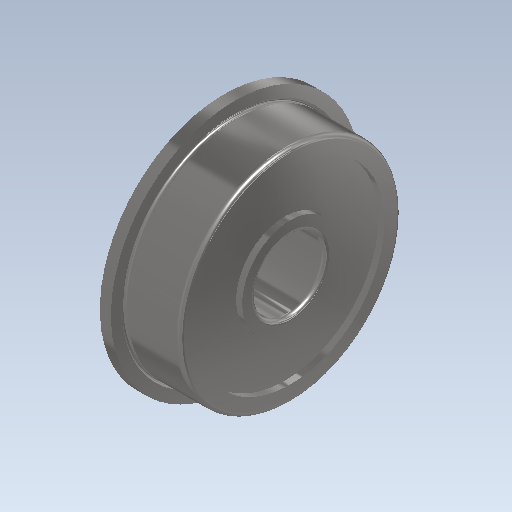
# Autodesk Inventor part: flange-bearing
Saved by Autodesk Inventor 2020 (Build 240168000, 168)
## iProperties
Part Number: flange-bearing
Material: Stainless Steel, 440C
Catalog Web Link: www.cadenas.de
Description: SFLC6 _ _ ZZ-Low Dust Raise Greased Ball Bearings - Double Shielded with Flange
Vendor: MISUMI
Document SubType Name: Modeling
Designer: partserver
Manufacturer: MISUMI
Mass: 12.691 g
Surface Area: 13.427 cm^2
Volume: 1.63755 cm^3
Density: 7.75 g/cm^3
Appearance: Semi-Polished
Category: PARTsolutions
Company: MISUMI
PSOL_IDENT_0: {$CADENAS_DATA\23d-libs\misumi\metric\12_bearing_holders\sflc673zz.prj},165 {VTYP=3D},{NB=SFLC625ZZ}
PSOL_IDENT_1: ,{LINA=SFLC625ZZ},{NN=SFLC6 _ _ ZZ},{DATE=30.10.2020 16:03:33},{GEOMDATE=06.08.2009 00:00:00},{VERSI
PSOL_IDENT_2: ON=},{LINEID=410},{WBVAR=},{WBNUMERIC=}  {NB=SFLC625ZZ},{LINA=SFLC625ZZ},{KT=DUMMY},{PN=SFLC625ZZ},{
PSOL_IDENT_3: TYPE=SFLC625ZZ},{MATR=440C Stainless Steel Equivalent},{HARDR=57 ~ 63HRC},{MATS=304 Stainless Steel}
PSOL_IDENT_4: ,{MATRE=440C Stainless Steel Equivalent},{MATC=304 Stainless Steel},{BN=625ZZ},{DD=5},{AA=4.120},{BB=
PSOL_IDENT_5: 1.200},{D=16},{B=5.0},{D1=18.0},{C=1.00},{RR=0.30},{CR=1470},{COR=540},{DS=7},{DDHH=14.0},{R=0.30},{
PSOL_IDENT_6: MASS=5.2}
NB: SFLC625ZZ
NN: SFLC6 _ _ ZZ
NT: Low Dust Raise Greased Ball Bearings - Double Shielded with Flange
NBSYN: $PN.
LINA: SFLC625ZZ
CATALOG: Misumi
PN: SFLC625ZZ
MATR: 440C Stainless Steel Equivalent
HARDR: 57 ~ 63HRC
MATS: 304 Stainless Steel
MATRE: 440C Stainless Steel Equivalent
MATC: 304 Stainless Steel
BN: 625ZZ
DD: 5
D: 16
B: 5
D1: 0
C: 1
RR: 0.3
CR: 1470
COR: 540
DS: 7
DDHH: 14
R: 0.3
MASS: 5.2
SUPPLIER: MISUMI
ARTICLENO: SFLC625ZZ
BOMINFO: SFLC625ZZ
CREATOR: CADENAS GmbH
Title: SFLC625ZZ
Author: Cadenas PARTsolutions
Comments: Low Dust Raise Greased Ball Bearings - Double Shielded with Flange
Autodesk Inventor part; units mm, degrees
ref_plane "YZ Plane" through (0, 0, 0) normal (1, 0, 0) x (0, 1, 0)
ref_plane "XZ Plane" through (0, 0, 0) normal (0, 1, 0) x (-1, 0, 0)
ref_plane "XY Plane" through (0, 0, 0) normal (0, 0, 1) x (1, 0, 0)
sketch "Sketch_2" plane through (0, 0, 0) normal (0, 0, 1) x (1, 0, 0)
  line L0 (5.25, -2.05) -> (-1, -2.05)
  arc A0 (-1, 1.45) -> (-0.625, 1.075) centre (-0.625, 1.45) ccw
  line L1 (-0.625, 1.075) -> (4.875, 1.075)
  arc A1 (4.875, 1.075) -> (5.25, 1.45) centre (4.875, 1.45) ccw
  line L2 (5.25, 1.45) -> (5.25, 2.325)
  line L3 (5.25, 2.325) -> (4.7, 2.325)
  line L4 (4.7, 2.325) -> (4.7, 6.45)
  line L5 (4.7, 6.45) -> (5, 6.45)
  line L6 (5, 6.45) -> (5, 9.2)
  line L7 (5, 9.2) -> (4, 9.2)
  line L8 (4, 9.2) -> (4, 8.2)
  arc A2 (3.75, 7.95) -> (4, 8.2) centre (4, 7.95) ccw
  line L9 (3.75, 7.95) -> (-0.625, 7.95)
  arc A3 (-0.625, 7.95) -> (-1, 7.575) centre (-0.625, 7.575) ccw
  line L10 (-1, 7.575) -> (-1, 6.45)
  line L11 (-1, 6.45) -> (-0.45, 6.45)
  line L12 (-0.45, 6.45) -> (-0.45, 2.325)
  line L13 (-0.45, 2.325) -> (-1, 2.325)
  line L14 (-1, 2.325) -> (-1, 1.45)
  line L15 (-1, 7.575) -> (-1, 8.599) construction
  dimension "d2" = 5
  dimension "d3" = 1
  constraints: 32 end point, 8 point on circle, 4 centre point, 1 tangent, 1 vertical
  measures "d2" distance from line of L15 L8.end
  measures "d3" distance of L6.end L7.end
revolve "Revolution1" add sketch "Sketch_2" angle 360 about axis through (5.25, -2.05, 0) along (1, 0, 0)
ref_plane "to_housing_XY" through (0, 0, 0) normal (1, 0, 0) x (0, 0, -1)
ref_plane "to_housing_YZ" through (0, 0, 0) normal (0, 0, -1) x (0, 1, 0)
ref_plane "to_housing_ZX" through (0, 0, 0) normal (0, 1, 0) x (1, 0, 0)
body "Solid1"
